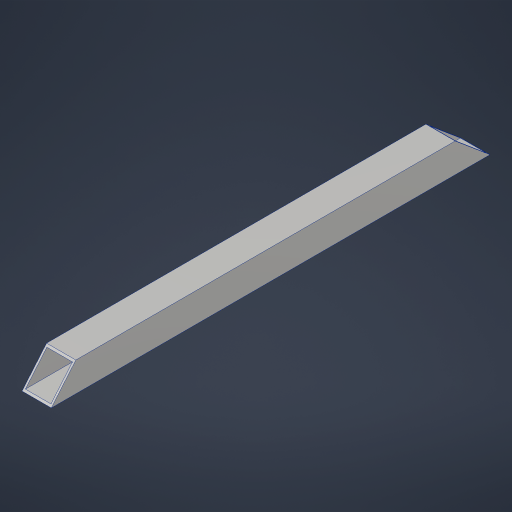
# Autodesk Inventor part: CL-002
Saved by Autodesk Inventor 2023.4 (Build 274418000, 418)
## iProperties
RuleStatus: InUse
Created: 2025-03-17
Part Number: CL-002
Material: Aluminum 6061
Document SubType Name: Modeling
Designer: dlangdon
Mass: 304.185 g
Surface Area: 718.547 cm^2
Volume: 112.661 cm^3
Density: 2.7 g/cm^3
Appearance: Aluminum - Flat
AfterDocNew0: SHOW
AfterDocOpen0: SHOW
Author: dlangdon
Autodesk Inventor part; units mm, degrees
ref_plane "YZ Plane" through (0, 0, 0) normal (1, 0, 0) x (0, 1, 0)
ref_plane "XZ Plane" through (0, 0, 0) normal (0, 1, 0) x (-1, 0, 0)
ref_plane "XY Plane" through (0, 0, 0) normal (0, 0, 1) x (1, 0, 0)
sketch "Sketch1" plane through (0, 0, 0) normal (0, 0, 1) x (1, 0, 0)
  line L0 (-12.7, -12.7) -> (12.7, -12.7)
  line L1 (12.7, -12.7) -> (12.7, 12.7)
  line L2 (12.7, 12.7) -> (-12.7, 12.7)
  line L3 (-12.7, 12.7) -> (-12.7, -12.7)
  line L4 (-12.7, -12.7) -> (12.7, 12.7) construction
  line L5 (12.7, -12.7) -> (-12.7, 12.7) construction
  line L6 (-11.1125, 11.1125) -> (11.1125, 11.1125)
  line L7 (11.1125, 11.1125) -> (11.1125, -11.1125)
  line L8 (11.1125, -11.1125) -> (-11.1125, -11.1125)
  line L9 (-11.1125, -11.1125) -> (-11.1125, 11.1125)
  point P0 (0, 0)
  dimension "width" = 25.4
  dimension "height" = 25.4
  dimension "thickness" = 1.5875
  constraints: 20 end point, 4 parallel, 2 midpoint, 2 perpendicular, 1 horizontal, 3 other
  measures "width" distance of L2.end L1.end
  measures "height" distance of L1.end L0.end
  measures "thickness" distance between parallel lines of L2 L6
extrude "Extrusion1" add sketch "Sketch1" along normal mid plane 381
sketch "Sketch2" plane through (12.7, -12.7, 190.5) normal (1, 0, 0) x (0, 0, -1)
  line L0 (0, 0) -> (157.42, 187.6059)
  line L1 (381, 0) -> (381, 25.4) projected
  line L2 (157.42, 187.6059) -> (381, 0)
  line L3 (0, 0) -> (0, 25.4) projected
  line L4 (381, 25.4) -> (0, 25.4) projected
  point P0 (190.5, 12.7)
  point P1 (350.7295, 25.4)
  point P2 (21.3131, 25.4)
  dimension "d5" = 40
  constraints: 4 end point, 1 coincident, 1 perpendicular
  measures "d5" angle of L3 L0
extrude "Extrusion2" cut sketch "Sketch2" against normal blind 25.4 contours L3 L4 L0 | L4 L1 L2
body "Solid1"
